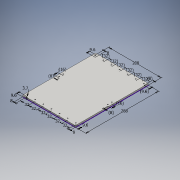
# Autodesk Inventor part: KrackenPlatedimensions
Saved by Autodesk Inventor 2016 (Build 200138000, 138)
## iProperties
Created: 2015-09-06
Part Number: KrackenPlatedimensions
Material: Generic
Document SubType Name: Modeling
Designer: Tim
Density: 1 g/cm^3
Appearance: Default
Author: Tim
Autodesk Inventor part; units mm, degrees
ref_plane "YZ Plane" through (0, 0, 0) normal (1, 0, 0) x (0, 1, 0)
ref_plane "XZ Plane" through (0, 0, 0) normal (0, 1, 0) x (-1, 0, 0)
ref_plane "XY Plane" through (0, 0, 0) normal (0, 0, 1) x (1, 0, 0)
sketch "Sketch1" plane through (0, 0, 0) normal (0, 0, 1) x (1, 0, 0)
  line L0 (104, -144) -> (-104, -144)
  line L1 (-104, -144) -> (-104, 144)
  line L2 (-104, 144) -> (104, 144)
  line L3 (104, 144) -> (104, -144)
  line L4 (104, -144) -> (-104, 144) construction
  line L5 (-104, -144) -> (104, 144) construction
  circle A0 centre (96, 134.4) radius 1.85
  circle A1 centre (64, 134.4) radius 1.85
  circle A2 centre (32, 134.4) radius 1.85
  circle A3 centre (0, 134.4) radius 1.85
  circle A4 centre (-32, 134.4) radius 1.85
  circle A5 centre (-64, 134.4) radius 1.85
  circle A6 centre (-96, 134.4) radius 1.85
  circle A7 centre (64, -134.4) radius 1.85
  circle A8 centre (32, -134.4) radius 1.85
  circle A9 centre (96, -134.4) radius 1.85
  circle A10 centre (0, -134.4) radius 1.85
  circle A11 centre (-32, -134.4) radius 1.85
  circle A12 centre (-96, -134.4) radius 1.85
  line L6 (104, 144) -> (-104, -144) construction
  line L7 (-104, 144) -> (104, -144) construction
  circle A13 centre (-64, -134.4) radius 1.85
  circle A14 centre (-96, 8) radius 1.85 projected
  circle A15 centre (-96, -8) radius 1.85 projected
  circle A16 centre (96, 8) radius 1.85 projected
  circle A17 centre (96, -8) radius 1.85 projected
  dimension "d0" = 208
  dimension "d1" = 288
  dimension "d13" = 3.7
  dimension "d14" = 32
  dimension "d15" = 32
  dimension "d16" = 9.6
  dimension "d17" = 8
  dimension "d18" = 8
  dimension "d19" = 9.6
  dimension "d20" = 8
  dimension "d21" = 9.6
  dimension "d22" = 9.6
  dimension "d23" = 8
  dimension "d24" = 16
  dimension "d25" = 8
  dimension "d26" = 16
  dimension "d27" = 8
  dimension "d28" = 32
  dimension "d29" = 32
  dimension "d30" = 32
  dimension "d31" = 32
  dimension "d32" = 32
  dimension "d33" = 32
  dimension "d34" = 32
  dimension "d35" = 32
  dimension "d36" = 32
  dimension "d37" = 32
  constraints: 16 end point, 2 parallel, 1 horizontal, 1 perpendicular
  measures "d0" distance of L2.start L2.end
  measures "d1" distance of L2.end L3.end
  measures "d13" diameter of A12
  measures "d14" distance of A13.centre A12.centre
  measures "d15" distance of A11.centre A13.centre
  measures "d16" distance from line of L0 A12.centre
  measures "d17" distance from line of L1 A12.centre
  measures "d18" distance from line of L1 A6.centre
  measures "d19" distance from line of L2 A6.centre
  measures "d20" distance from line of L3 A0.centre
  measures "d21" distance from line of L2 A0.centre
  measures "d22" distance from line of L0 A9.centre
  measures "d23" distance from line of L3 A9.centre
  measures "d24" distance of A14.centre A15.centre
  measures "d25" distance from line of A15.centre L1
  measures "d26" distance of A16.centre A17.centre
  measures "d27" distance from line of L3 A17.centre
  measures "d28" distance of A7.centre A9.centre
  measures "d29" distance of A7.centre A8.centre
  measures "d30" distance of A8.centre A10.centre
  measures "d31" distance of A10.centre A11.centre
  measures "d32" distance of A6.centre A5.centre
  measures "d33" distance of A4.centre A5.centre
  measures "d34" distance of A4.centre A3.centre
  measures "d35" distance of A3.centre A2.centre
  measures "d36" distance of A2.centre A1.centre
  measures "d37" distance of A1.centre A0.centre
extrude "Extrusion5" add sketch "Sketch1" along normal blind 6
body "Solid5"
